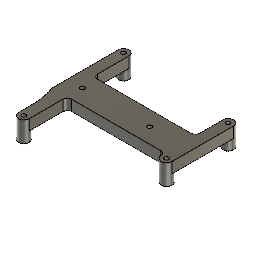
arduino-uno-mount (Autodesk Fusion 360 design; units mm, degrees)
Autodesk Fusion 360 part; units mm, degrees
sketch "Sketch1" plane through (0, 0, 0) normal (0, 0, 1) x (1, 0, 0)
  line L0 (52, 35) -> (52, -35) construction
  line L1 (-52, -32) -> (-49, -32) construction
  line L2 (-34.5, 7) -> (-34.5, -7)
  line L3 (-34.5, -7) -> (34.5, -7)
  line L4 (34.5, -7) -> (34.5, 7)
  line L5 (34.5, 7) -> (-34.5, -7) construction
  line L6 (-34.5, 7) -> (34.5, -7) construction
  line L7 (-51.5, -32) -> (-46.5, -32)
  line L8 (31.5, 7) -> (26.5, 7)
  line L9 (0, 0) -> (15.5, 0) construction
  line L10 (0, 0) -> (-15.5, 0) construction
  circle A0 centre (15.5, 0) radius 1
  circle A1 centre (15.5, 0) radius 2
  circle A2 centre (-15.5, 0) radius 1
  circle A3 centre (-15.5, 0) radius 2
  line L11 (0, 0) -> (93.1232, 0) construction
  line L12 (-34.5, 7) -> (34.5, 7)
  line L13 (34.5, 0) -> (34.5, -8.75) construction
  line L14 (34.5, -8.75) -> (29.5, -8.75)
  line L15 (29.5, -8.75) -> (29.5, -7)
  line L16 (29.5, -7) -> (34.5, -7)
  line L17 (34.5, -7) -> (34.5, -8.75)
  line L18 (34.5, -8.75) -> (32, -8.75) construction
  circle A4 centre (32, -8.75) radius 2.5
  circle A5 centre (32, -8.75) radius 0.95
  line L19 (32, -8.75) -> (-18, -8.75) construction
  line L20 (32, -8.75) -> (-20, -8.75) construction
  line L21 (-15.5, 0) -> (-15.5, -24.5) construction
  line L22 (-15.5, -24.5) -> (-43.4212, -24.5) construction
  line L23 (-18, -8.75) -> (-18, -24.5) construction
  line L24 (-20, -8.75) -> (-20.05, 23.5) construction
  circle A6 centre (-20.05, 23.5) radius 2.5
  circle A7 centre (-18, -24.5) radius 2.5
  line L25 (-20.5, -24.5) -> (-15.5, -24.5)
  line L26 (-15.5, -24.5) -> (-15.5, -7)
  line L27 (-15.5, -7) -> (-20.5, -7)
  line L28 (-20.5, -7) -> (-20.5, -24.5)
  line L29 (-20.5, 7) -> (-15.5, 7)
  circle A8 centre (-18, -24.5) radius 0.95
  circle A9 centre (-20.05, 23.5) radius 0.95
  line L30 (34.5, 0) -> (34.5, 19.75) construction
  line L31 (34.5, 19.75) -> (29.5, 19.75)
  line L32 (29.5, 19.75) -> (29.5, 7)
  line L33 (29.5, 7) -> (34.5, 7)
  line L34 (34.5, 7) -> (34.5, 19.75)
  circle A10 centre (32.0009, 19.6821) radius 2.5
  circle A11 centre (32.0009, 19.6821) radius 0.95
  line L35 (-20.05, 23.5) -> (-19.1, 23.5015) construction
  line L36 (-20.05, 23.5) -> (-27.9475, 23.4878) construction
  line L37 (-22.55, 23.4961) -> (-17.55, 23.4961)
  line L38 (-17.55, 23.4961) -> (-17.55, 7)
  line L39 (-17.55, 7) -> (-22.55, 7)
  line L40 (-22.55, 7) -> (-22.55, 23.4961)
  line L41 (-22.55, 7) -> (-22.55, -8.8394)
  dimension "d19" = 14
  dimension "d28" = 15.5
  dimension "d29" = 15.5
  dimension "d30" = 2
  dimension "d31" = 4
  dimension "d32" = 2
  dimension "d33" = 4
  dimension "d60" = 69
  dimension "d62" = 8.75
  dimension "d64" = 5
  dimension "d65" = 2.5
  dimension "d66" = 5
  dimension "d67" = 1.9
  dimension "d68" = 50
  dimension "d69" = 52
  dimension "d72" = 24.5
  dimension "d73" = 5
  dimension "d74" = 5
  dimension "d75" = 5
  dimension "d77" = 1.9
  dimension "d78" = 1.9
  dimension "d99" = 19.75
  dimension "d100" = 5
  dimension "d101" = 5
  dimension "d102" = 1.9
  dimension "d131" = 5
  dimension "d140" = 32.25
  constraint coincident L9.start L10.start
  constraint parallel L2 L4
  constraint coincident L5 L9.start
  constraint coincident L6 L9.start
  constraint coincident L1 L7.start
  constraint horizontal L8
  constraint horizontal L9
  constraint horizontal L10
  constraint coincident L9.end A0.centre
  constraint concentric A0 A1
  constraint coincident L10.end A2.centre
  constraint concentric A2 A3
  constraint horizontal L11
  constraint perpendicular L4 L12
  constraint midpoint L4 L13.start
  constraint perpendicular L11 L13
  constraint horizontal L14
  constraint vertical L15
  constraint horizontal L16
  constraint vertical L17
  constraint perpendicular L13 L18
  constraint coincident L18.end A4.centre
  constraint concentric A4 A5
  constraint parallel L14 L19
  constraint parallel L18 L20
  constraint perpendicular L10 L21
  constraint perpendicular L21 L22
  constraint coincident L22 L23.end
  constraint perpendicular L22 L23
  constraint coincident L24.end A6.centre
  constraint coincident L23.end A7.centre
  constraint horizontal L25
  constraint vertical L26
  constraint horizontal L27
  constraint vertical L28
  constraint coincident A7 L25.start
  constraint coincident L22 L25.start
  constraint horizontal L29
  constraint concentric A7 A8
  constraint concentric A6 A9
  constraint perpendicular L11 L30
  constraint horizontal L31
  constraint vertical L32
  constraint horizontal L33
  constraint vertical L34
  constraint coincident L30.end A10
  constraint concentric A10 A11
  constraint coincident A9 L35.end
  constraint perpendicular L24 L35
  constraint perpendicular L24 L36
  constraint horizontal L37
  constraint vertical L38
  constraint horizontal L39
  constraint vertical L40
  constraint coincident A6 L37.start
  constraint coincident L36 L37.start
  constraint perpendicular L3 L41
  measures "d19" distance of L2.start L2.end
  measures "d28" distance of L9.start L9.end
  measures "d29" distance of L9.start L10.end
  measures "d30" diameter of A0
  measures "d31" diameter of A1
  measures "d32" diameter of A2
  measures "d33" diameter of A3
  measures "d60" distance of L4.end L2.start
  measures "d62" distance of L13.start L13.end
  measures "d64" distance of L13.end L14.end
  measures "d65" distance of L13.end L18.end
  measures "d66" diameter of A4
  measures "d67" diameter of A5
  measures "d68" distance of L18.end L19.end
  measures "d69" distance of L18.end L20.end
  measures "d72" distance of L10.end L21.end
  measures "d73" diameter of A6
  measures "d74" diameter of A7
  measures "d75" distance of L25.start L21.end
  measures "d77" diameter of A8
  measures "d78" diameter of A9
  measures "d99" distance of L13.start L30.end
  measures "d100" distance of L30.end L31.end
  measures "d101" diameter of A10
  measures "d102" diameter of A11
  measures "d131" distance of L37.start L37.end
  measures "d140" vertical distance of L20.end L24.end
extrude "Extrude6" add sketch "Sketch1" along normal blind 5 contours L3 L15 L16 A4 | L3 L14 L16 A4 A5 | L14 A4 A5 | L8 L12 L31 L32 L33 L34 A10 | L3 L16 L17 A4 | L31 A10 A11 | L31 L34 A10 A11 | L34 A10 makes body 1 at (34.4969, -8.8746, 3.3333) makes body 2 at (31.9766, 10.9116, 5)
extrude "Extrude9" add sketch "Sketch1" against normal blind 5 contours L31 L34 A10 A11 | A6 A9 L37 | A6 A9 L37 | A7 L25 A8 | A7 L25 A8 | L3 L16 A4 | L3 L14 L16 A4 A5 | L14 A4 A5 | L31 A10 A11 bodies 1 2 makes body 3 at (-15.5031, -24.6246, -3.3333) makes body 4 at (-22.5471, 23.6208, -3.3333)
extrude "Extrude7" add sketch "Sketch1" along normal blind 5 contours L12 A6 L29 L38 L39 L40 | L3 L4 L8 L12 L16 A4 L27 L29 L33 L39 L41 | A6 A9 L37 | A6 A9 L37 | L3 A7 L26 L27 L28 | A7 L25 A8 | A7 L25 A8 | L3 L16 A4 | A1 | A3 bodies 1 4 2 3
extrude "Extrude8" cut sketch "Sketch1" along normal blind 2 contours A1 | A3 bodies 1
fillet "Fillet25" radius 0.5 6 edges at (-22.3808, 24.404, -5) (-20.3308, -23.596, -5) (29.6692, -7.846, -5) (29.6701, 20.5862, -5) (13.6353, -0.7232, 0) (-17.3647, -0.7232, 0) on bodies 1 2
fillet "Fillet28" radius 33 1 edges at (-20.5, -7, 2.5) on bodies 1
fillet "Fillet29" radius 0.25 4 edges at (-20.9357, 23.1565, -5) (-18.8857, -24.8435, -5) (31.1143, -9.0935, -5) (31.1152, 19.3386, -5) on bodies 1 2
fillet "Fillet30" radius 2 4 edges at (-17.55, 7, 2.5) (-15.5, -7, 2.5) (29.5, 7, 2.5) (29.5, -7, 2.5) on bodies 1
equation "mholefromtop = 47.5 mm"
equation "topleft = 19 mm"
equation "topbetween = 62 mm"
equation "topdown = 3 mm"
equation "rightin = 5 mm"
equation "corner = 3 mm"
equation "outerhole = 5 mm"
equation "m2hole = 1.9 mm"
equation "barwidth = 5 mm"
equation "d28 = ( 31 / 2 ) * 1 mm"
equation "d29 = ( 31 / 2 ) * 1 mm"
equation "d60 = basewidth"
equation "basewidth = 69 mm"
equation "d62 = ( 28.5 / 2 - 5.5 ) * 1 mm"
equation "d64 = barwidth"
equation "d65 = barwidth / 2"
equation "d66 = barwidth"
equation "d67 = m2hole"
equation "d72 = ( ( 48 / 2 ) * 1 ) * 1 mm + 0.5 mm"
equation "d73 = outerhole"
equation "d77 = m2hole"
equation "d78 = m2hole"
equation "d99 = ( 28.5 / 2 + 5.5 ) * 1 mm"
equation "d102 = m2hole"
equation "armwidth = 7 mm"
